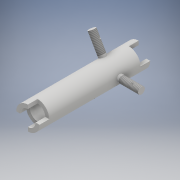
# Autodesk Inventor part: ObererRührerHalter
Saved by Autodesk Inventor 2017 (Build 210142000, 142)
## iProperties
Created: 2019-06-23
Part Number: ObererRührerHalter
Material: Generic
Document SubType Name: Modeling
Designer: Ole Simmering
Density: 1 g/cm^3
Appearance: Default
Author: Ole Simmering
Autodesk Inventor part; units mm, degrees
sketch "Sketch1" plane through (0, 0, 0) normal (0, 1, 0) x (-1, 0, 0)
  circle A0 centre (0, 0) radius 4
  circle A1 centre (0, 0) radius 6
  dimension "d0" = 8
  dimension "d1" = 12
  constraints: 2 centre point, 2 coincident
  measures "d0" diameter of A0
  measures "d1" diameter of A1
extrude "Extrusion1" add sketch "Sketch1" along normal blind 47
sketch "Sketch2" plane through (0, 47, 0) normal (0, 1, 0) x (1, 0, 0)
  circle A0 centre (0, 0) radius 6 construction
  arc A1 (-6, 0) -> (0, -6) centre (0, 0) ccw
  circle A2 centre (0, 0) radius 4 construction
  arc A3 (-4, 0) -> (0, -4) centre (0, 0) ccw
  line L0 (0, -6) -> (0, -4)
  line L1 (-4, 0) -> (-6, 0)
  line L2 (4, 0) -> (6, 0)
  arc A4 (6, 0) -> (0, 6) centre (0, 0) ccw
  arc A5 (4, 0) -> (0, 4) centre (0, 0) ccw
  line L3 (0, 6) -> (0, 4)
  dimension "d6" = 360
  constraints: 8 end point, 8 point on circle, 4 centre point, 3 coincident, 2 vertical alignment, 1 perpendicular, 1 vertical, 23 other
extrude "Extrusion2" add sketch "Sketch2" along normal blind 5
ref_plane "Work Plane5" through (0, 37, 0) normal (0, -1, 0) x (1, 0, 0)
ref_plane "Work Plane1" through (0, 23.5, 0) normal (0, 1, 0) x (1, 0, 0)
mirror "Mirror1" about plane through (0, 23.5, 0) normal (0, 1, 0) of "Extrusion2"
sketch "Sketch3" plane through (0, 37, 0) normal (0, -1, 0) x (1, 0, 0)
  arc A0 (-6, 0) -> (0, -6) centre (0, 0) ccw construction
  line L0 (0, -6) -> (0, -4) construction
  arc A1 (-4, 0) -> (0, -4) centre (0, 0) ccw construction
  line L1 (-4, 0) -> (-6, 0) construction
  line L2 (-6, 0) -> (-4, 0) construction
  arc A2 (0, 4) -> (-4, 0) centre (0, 0) ccw construction
  line L3 (0, 4) -> (0, 6) construction
  arc A3 (0, 6) -> (-6, 0) centre (0, 0) ccw construction
  arc A4 (4, 0) -> (0, 4) centre (0, 0) ccw construction
  line L4 (4, 0) -> (6, 0) construction
  arc A5 (6, 0) -> (0, 6) centre (0, 0) ccw construction
  line L5 (0, 6) -> (0, 4) construction
  line L6 (0, -4) -> (0, -6) construction
  arc A6 (0, -6) -> (6, 0) centre (0, 0) ccw construction
  line L7 (6, 0) -> (4, 0) construction
  arc A7 (0, -4) -> (4, 0) centre (0, 0) ccw construction
  line L8 (6, 0) -> (11.7956, 0) construction
  line L9 (0, 0) -> (-6.4031, -11.0905) construction
  line L10 (0, 0) -> (-6.364, 11.0227) construction
  dimension "d10" = 120
  dimension "d11" = 120
  constraints: 22 end point, 16 point on circle, 8 centre point, 1 horizontal
  measures "d10" angle of L8 L9
  measures "d11" angle of L10 L8
ref_plane "Work Plane2" through (6, 37, 0) normal (1, 0, 0) x (0, 1, 0)
sketch "Sketch4" plane through (6, 37, 0) normal (1, 0, 0) x (0, 1, 0)
  line L0 (-42, -6) -> (-42, 0) construction
  circle A0 centre (-0.5, 0) radius 1.75
  point P0 (-37, 0)
  dimension "d12" = 41.5
  dimension "d38" = 3.5
  constraints: 1 centre point, 1 coincident
  measures "d12" distance from line of L0 point (-0.5, 0)
  measures "d38" diameter of A0
extrude "Extrusion3" add sketch "Sketch4" along normal blind 11 and the other way blind 0.5
pattern_circular "Circular Pattern1" count 3 over 360 about axis through (0, 0, 0) along (0, 1, 0) of "Extrusion3"
thread "Thread1" size "M3.5x0.6" class "6g" standard "ANSI Metric M Profile" length 10
thread "Thread2" size "M3.5x0.6" class "6g" standard "ANSI Metric M Profile" length 10
thread "Thread3" size "M3.5x0.6" class "6g" standard "ANSI Metric M Profile" length 10
ref_plane "Work Plane3" through (-6.5, 36.5, 11.2583) normal (-0.5, 0, 0.866) x (0.866, 0, 0.5)
sketch "Sketch6" plane through (-6.5, 36.5, 11.2583) normal (-0.5, 0, 0.866) x (0.866, 0, 0.5)
  line L0 (0, 0) -> (-3.1225, -1.8028) construction
  line L1 (0, 0) -> (0, 3.8525) construction
  point P0 (0, -36.5)
  point P1 (-1.7321, -1)
  dimension "d27" = 120
  constraints: 4 end point, 1 point on line, 1 vertical
  measures "d27" angle of L0 L1
ref_plane "Work Plane4" through (-8, 35.5, 10.3923) normal (-0.75, -0.5, -0.433) x (0.5547, -0.8321, 0)
sketch "Sketch7" plane through (-8, 35.5, 10.3923) normal (-0.75, -0.5, -0.433) x (0.5547, -0.8321, 0)
  point P0 (33.9754, -3.723)
  point P1 (0, 0)
hole "Hole1" at (-8, 35.5, 10.3923) direction (0.75, 0.5, 0.433) diameter 1 end through all
pattern_circular "Circular Pattern2" count 3 over 360 about axis through (0, 0, 0) along (0, 1, 0) of "Hole1"
body "Solid1"
